y_bearing_holder (Autodesk Fusion 360 design; units mm, degrees)
Autodesk Fusion 360 part; units mm, degrees
sketch "Sketch1" plane through (0, 0, 0) normal (0, 0, 1) x (1, 0, 0)
  line L0 (-7.6, 0) -> (-12.6, 0)
  line L1 (-12.6, 0) -> (-25, 6)
  line L2 (-25, 6) -> (-25, 13)
  line L3 (-25, 13) -> (15, 13)
  line L4 (15, 13) -> (15, 6)
  line L5 (15, 6) -> (12.6, 0)
  line L6 (12.6, 0) -> (7.6, 0)
  arc A0 (7.6, 0) -> (-7.6, 0) centre (0, 0) ccw
  dimension "d1" = 15.2
  dimension "d2" = 5
  dimension "d3" = 7
  dimension "d4" = 13
  dimension "d5" = 40
  dimension "d6" = 15
  constraint coincident A0.centre origin
  constraint horizontal L0
  constraint perpendicular L0 L2
  constraint perpendicular L2 L3
  constraint perpendicular L3 L4
  constraint perpendicular L4 L6
  constraint horizontal L0.start L6.end
  constraint horizontal A0.centre L0.start
  constraint equal L0 L6
  constraint horizontal L1.end L4.end
  measures "d1" diameter of A0
  measures "d2" distance of L5.end L6.end
  measures "d3" distance of L3.end L4.end
  measures "d4" distance of A0.centre L3
  measures "d5" distance of L2.end L3.end
  measures "d6" distance of A0.centre L4
extrude "Extrude1" add sketch "Sketch1" along normal blind 30
sketch "Sketch2" plane through (0, 13, 0) normal (0, 1, 0) x (-1, 0, 0)
  line L0 (-15, 0) -> (25, 0)
  line L1 (25, 0) -> (25, 30)
  line L2 (25, 30) -> (-15, 30)
  line L3 (-15, 30) -> (-15, 0)
  circle A0 centre (19.5, 6) radius 2.1
  circle A1 centre (-4.5, 6) radius 2.1
  circle A2 centre (19.5, 24) radius 3.6
  circle A3 centre (-4.5, 24) radius 3.6
  circle A4 centre (-4.5, 24) radius 2.1
  circle A5 centre (19.5, 24) radius 2.1
  circle A6 centre (19.5, 6) radius 3.6
  circle A7 centre (-4.5, 6) radius 3.6
  line L4 (19.5, 6) -> (-4.5, 24) construction
  point P0 (7.5, 15)
  dimension "d9" = 4.2
  dimension "d10" = 7.2
  dimension "d11" = 24
  dimension "d12" = 18
  dimension "d13" = 17.5
  dimension "d14" = 15
  constraint concentric A3 A4
  constraint concentric A2 A5
  constraint concentric A0 A6
  constraint concentric A1 A7
  constraint equal A0 A1
  constraint equal A1 A4
  constraint equal A4 A5
  constraint equal A6 A7
  constraint equal A3 A7
  constraint equal A2 A3
  constraint vertical A0.centre A2.centre
  constraint vertical A1.centre A3.centre
  constraint horizontal A2.centre A3.centre
  constraint horizontal A1.centre A0.centre
  constraint coincident A0.centre A6.centre
  constraint coincident A3.centre A4.centre
  constraint midpoint L4 P0
  measures "d9" diameter of A0
  measures "d10" diameter of A7
  measures "d11" distance of A0.centre A1.centre
  measures "d12" distance of A2.centre A0.centre
  measures "d13" distance of L1 P0
  measures "d14" distance of L2 P0
extrude "Extrude2" cut sketch "Sketch2" against normal through all contours A0 | A1 | A4 | A5
sketch "Sketch3" plane through (0, 0, 30) normal (0, 0, 1) x (1, 0, 0)
  line L0 (7.6, 0) -> (12.6, 0)
  line L1 (12.6, 0) -> (15, 6)
  line L2 (15, 6) -> (15, 13)
  line L3 (15, 13) -> (-25, 13)
  line L4 (-25, 13) -> (-25, 6)
  line L5 (-25, 6) -> (-12.6, 0)
  line L6 (-12.6, 0) -> (-7.6, 0)
  arc A0 (7.6, 0) -> (-7.6, 0) centre (0, 0) ccw
  line L7 (-7.6, 0) -> (-5, 0)
  line L8 (5, 0) -> (7.6, 0)
  arc A1 (5, 0) -> (-5, 0) centre (0, 0) ccw
  dimension "d19" = 10
  constraint concentric A0 A1
  constraint coincident L6.end A0.end
  constraint parallel L6 L7
  constraint coincident L0.start A0.start
  constraint parallel L0 L8
  measures "d19" diameter of A1
extrude "Extrude4" add sketch "Sketch3" against normal blind 2.9 contours A0 L7 L8 A1
extrude "Extrude5" add sketch "Sketch3" along normal blind 2.9 from surface at -30 contours A0 L7 L8 A1
extrude "Extrude3" cut sketch "Sketch2" along normal blind 11 from surface at -13 contours A2 | A3 | A6 | A7
sketch "Sketch4" plane through (0, 0, 30) normal (0, 0, 1) x (1, 0, 0)
  line L0 (5, 0) -> (12.6, 0)
  line L1 (12.6, 0) -> (15, 6)
  line L2 (15, 6) -> (15, 13)
  line L3 (15, 13) -> (-25, 13)
  line L4 (-25, 13) -> (-25, 6)
  line L5 (-25, 6) -> (-12.6, 0)
  line L6 (-12.6, 0) -> (-5, 0)
  arc A0 (5, 0) -> (-5, 0) centre (0, 0) ccw
  line L7 (-8, 0) -> (-8.89, 3.195)
  line L8 (-8.4, 5.8) -> (-5.4, 9.8)
  line L9 (-3, 11) -> (3, 11)
  line L10 (5.4, 9.8) -> (8.4, 5.8)
  line L11 (8.89, 3.195) -> (8, 0)
  arc A1 (-8.4, 5.8) -> (-8.89, 3.195) centre (-6, 4) ccw
  arc A2 (-3, 11) -> (-5.4, 9.8) centre (-3, 8) ccw
  arc A3 (5.4, 9.8) -> (3, 11) centre (3, 8) ccw
  arc A4 (8.89, 3.195) -> (8.4, 5.8) centre (6, 4) ccw
  line L12 (-9.9266, -0.5367) -> (-10.8166, 2.6583)
  arc A5 (-10, 7) -> (-10.8166, 2.6583) centre (-6, 4) ccw
  line L13 (-10, 7) -> (-7, 11)
  arc A6 (-3, 13) -> (-7, 11) centre (-3, 8) ccw
  line L14 (-3, 13) -> (3, 13)
  arc A7 (7, 11) -> (3, 13) centre (3, 8) ccw
  line L15 (7, 11) -> (10, 7)
  arc A8 (10.8166, 2.6583) -> (10, 7) centre (6, 4) ccw
  line L16 (10.8166, 2.6583) -> (9.9266, -0.5367)
  dimension "d25" = 2
  dimension "d26" = 3
  dimension "d27" = 6
  dimension "d28" = 6
  dimension "d29" = 4
  dimension "d30" = 3
  dimension "d31" = 8
  dimension "d32" = 8
  dimension "d33" = 3
  dimension "d34" = -2
  constraint parallel L6 L9
  constraint tangent L7 A1
  constraint tangent L8 A1
  constraint tangent L8 A2
  constraint tangent L9 A2
  constraint equal A1 A2
  constraint tangent L9 A3
  constraint tangent L10 A3
  constraint equal A1 A3
  constraint tangent L10 A4
  constraint tangent L11 A4
  constraint equal A1 A4
  constraint horizontal A1.centre A4.centre
  constraint coincident L6 L7.start
  constraint coincident L0 L11.end
  measures "d25" distance of L3 L9
  measures "d26" radius of A1
  measures "d27" horizontal distance of A0.centre A1.centre
  measures "d28" horizontal distance of A0.centre A4.centre
  measures "d29" distance of L0 A4.centre
  measures "d30" horizontal distance of A0.centre A2.centre
  measures "d31" distance of A0.centre L7.start
  measures "d32" distance of A0.centre L11.end
  measures "d33" horizontal distance of A0.centre A3.centre
extrude "Extrude6" cut sketch "Sketch4" along normal mid plane 4 from surface at -15 contours L0 L3 L6 L7 L8 L9 L10 L11 A1 A2 A3 A4 L12 A5 L13 A6 L14 A7 L15 A8 L16
fillet "Fillet1" radius 1 4 edges at (-8, 0, 15) (8, 0, 15) (-3, 13, 15) (3, 13, 15)
fillet "Fillet2" radius 5 4 edges at (-12.6, 0, 15) (12.6, 0, 15) (15, 6, 15) (-25, 6, 15)
equation "d13 = ( 35 / 2 ) * 1 mm"
equation "d28 = d27"
equation "d32 = d31"
equation "d33 = d30"
